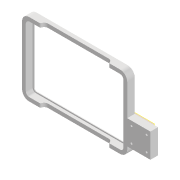
# Autodesk Inventor part: 20_Cube_Insert_Linear_Stage_NEMA11_china_wellplatemount
Saved by Autodesk Inventor 2022 (Build 260153000, 153)
## iProperties
Created: 2022-01-15
Part Number: 20_Cube_Insert_Linear_Stage_NEMA11_china_wellplatemount
Material: Generisch
Document SubType Name: Modeling
Designer: diederichbenedict
Density: 1 g/cm^3
Appearance: Vorgabe
Author: diederichbenedict
Autodesk Inventor part; units mm, degrees
ref_plane "YZ Plane" through (0, 0, 0) normal (1, 0, 0) x (0, 1, 0)
ref_plane "XZ Plane" through (0, 0, 0) normal (0, 1, 0) x (-1, 0, 0)
ref_plane "XY Plane" through (0, 0, 0) normal (0, 0, 1) x (1, 0, 0)
ref_plane "Arbeitsebene1" through (-6.2499, 0, 0) normal (0, 0, 1) x (1, 0, 0)
sketch "Skizze1" plane through (-6.2499, 0, 0) normal (0, 0, 1) x (1, 0, 0)
  line L0 (21.2499, 26.0506) -> (21.2499, 58.2506) projected
  line L1 (21.2499, 58.2506) -> (-8.7501, 58.2506) projected
  line L2 (-8.7501, 58.2506) -> (-8.7501, 26.0506) projected
  line L3 (-8.7501, 26.0506) -> (21.2499, 26.0506) projected
  circle A0 centre (16.2499, 32.1506) radius 1.25 projected
  circle A1 centre (-3.7501, 32.1506) radius 1.25 projected
  circle A2 centre (-3.7501, 52.1506) radius 1.25 projected
  circle A3 centre (16.2499, 52.1506) radius 1.25 projected
  circle A4 centre (13.7499, 38.0506) radius 3.25 projected
  circle A5 centre (13.7499, 46.2506) radius 3.25 projected
  circle A6 centre (-1.2501, 38.0506) radius 3.25 projected
  circle A7 centre (-1.2501, 46.2506) radius 3.25 projected
  line L4 (-67.7501, 103.2266) -> (-67.7501, 101.9266) construction
  line L5 (-18.7501, 103.2266) -> (-67.7501, 103.2266) construction
  arc A8 (-15.2501, 99.7266) -> (-18.7501, 103.2266) centre (-18.7501, 99.7266) ccw construction
  line L6 (-15.2501, 22.1266) -> (-15.2501, 99.7266) construction
  arc A9 (-18.7501, 18.6266) -> (-15.2501, 22.1266) centre (-18.7501, 22.1266) ccw construction
  line L7 (-67.7501, 18.6266) -> (-18.7501, 18.6266) construction
  line L8 (-67.7501, 19.9266) -> (-67.7501, 18.6266) construction
  line L9 (-23.4028, 19.9266) -> (-67.7501, 19.9266) construction
  arc A10 (-23.4028, 19.9266) -> (-21.8472, 20.571) centre (-23.4028, 22.1266) ccw construction
  line L10 (-17.1945, 25.2237) -> (-21.8472, 20.571) construction
  arc A11 (-17.1945, 25.2237) -> (-16.5501, 26.7793) centre (-18.7501, 26.7793) ccw construction
  line L11 (-16.5501, 95.0739) -> (-16.5501, 26.7793) construction
  arc A12 (-16.5501, 95.0739) -> (-17.1945, 96.6296) centre (-18.7501, 95.0739) ccw construction
  line L12 (-21.8472, 101.2823) -> (-17.1945, 96.6296) construction
  arc A13 (-21.8472, 101.2823) -> (-23.4028, 101.9266) centre (-23.4028, 99.7266) ccw construction
  line L13 (-67.7501, 101.9266) -> (-23.4028, 101.9266) construction
  arc A14 (-18.7501, 18.2266) -> (-14.8501, 22.1266) centre (-18.7501, 22.1266) ccw construction
  line L14 (-14.8501, 22.1266) -> (-14.8501, 99.7266) construction
  line L15 (-18.7501, 103.6266) -> (-68.1501, 103.6266) construction
  line L16 (-68.1501, 103.6266) -> (-68.1501, 101.5266) construction
  line L17 (-68.1501, 101.5266) -> (-23.4028, 101.5266) construction
  arc A15 (-22.13, 100.9994) -> (-23.4028, 101.5266) centre (-23.4028, 99.7266) ccw construction
  line L18 (-22.13, 100.9994) -> (-17.4773, 96.3467) construction
  arc A16 (-16.9501, 95.0739) -> (-17.4773, 96.3467) centre (-18.7501, 95.0739) ccw construction
  line L19 (-16.9501, 95.0739) -> (-16.9501, 26.7793) construction
  arc A17 (-17.4773, 25.5065) -> (-16.9501, 26.7793) centre (-18.7501, 26.7793) ccw construction
  line L20 (-17.4773, 25.5065) -> (-22.13, 20.8538) construction
  arc A18 (-23.4028, 20.3266) -> (-22.13, 20.8538) centre (-23.4028, 22.1266) ccw construction
  line L21 (-23.4028, 20.3266) -> (-68.1501, 20.3266) construction
  line L22 (-68.1501, 20.3266) -> (-68.1501, 18.2266) construction
  line L23 (-68.1501, 18.2266) -> (-18.7501, 18.2266) construction
  arc A19 (-18.7501, 18.2266) -> (-14.8501, 22.1266) centre (-18.7501, 22.1266) ccw construction
  line L24 (-14.8501, 22.1266) -> (-14.8501, 99.7266) construction
  arc A20 (-14.8501, 99.7266) -> (-18.7501, 103.6266) centre (-18.7501, 99.7266) ccw construction
  line L25 (-89.5501, 101.9266) -> (-89.5501, 103.2266) construction
  line L26 (-138.8501, 101.9266) -> (-89.5501, 101.9266) construction
  arc A21 (-138.8501, 101.9266) -> (-140.7501, 100.0266) centre (-138.8501, 100.0266) ccw construction
  line L27 (-140.7501, 21.8266) -> (-140.7501, 100.0266) construction
  arc A22 (-140.7501, 21.8266) -> (-138.8501, 19.9266) centre (-138.8501, 21.8266) ccw construction
  line L28 (-89.5501, 19.9266) -> (-138.8501, 19.9266) construction
  line L29 (-89.5501, 18.6266) -> (-89.5501, 19.9266) construction
  line L30 (-138.5501, 18.6266) -> (-89.5501, 18.6266) construction
  arc A23 (-142.0501, 22.1266) -> (-138.5501, 18.6266) centre (-138.5501, 22.1266) ccw construction
  line L31 (-142.0501, 99.7266) -> (-142.0501, 22.1266) construction
  arc A24 (-138.5501, 103.2266) -> (-142.0501, 99.7266) centre (-138.5501, 99.7266) ccw construction
  line L32 (-89.5501, 103.2266) -> (-138.5501, 103.2266) construction
  arc A25 (-138.5501, 103.6266) -> (-142.4501, 99.7266) centre (-138.5501, 99.7266) ccw construction
  line L33 (-142.4501, 99.7266) -> (-142.4501, 22.1266) construction
  arc A26 (-142.4501, 22.1266) -> (-138.5501, 18.2266) centre (-138.5501, 22.1266) ccw construction
  line L34 (-138.5501, 18.2266) -> (-89.1501, 18.2266) construction
  line L35 (-89.1501, 18.2266) -> (-89.1501, 20.3266) construction
  line L36 (-89.1501, 20.3266) -> (-138.8501, 20.3266) construction
  arc A27 (-140.3501, 21.8266) -> (-138.8501, 20.3266) centre (-138.8501, 21.8266) ccw construction
  line L37 (-140.3501, 21.8266) -> (-140.3501, 100.0266) construction
  arc A28 (-138.8501, 101.5266) -> (-140.3501, 100.0266) centre (-138.8501, 100.0266) ccw construction
  line L38 (-138.8501, 101.5266) -> (-89.1501, 101.5266) construction
  line L39 (-89.1501, 101.5266) -> (-89.1501, 103.6266) construction
  line L40 (-89.1501, 103.6266) -> (-138.5501, 103.6266) construction
  line L41 (-68.6501, 104.1266) -> (-18.7501, 104.1266)
  arc A29 (-14.3501, 99.7266) -> (-18.7501, 104.1266) centre (-18.7501, 99.7266) ccw
  line L42 (-14.3501, 99.7266) -> (-14.3501, 22.1266)
  arc A30 (-18.7501, 17.7266) -> (-14.3501, 22.1266) centre (-18.7501, 22.1266) ccw
  line L43 (-18.7501, 17.7266) -> (-68.6501, 17.7266)
  line L44 (-68.6501, 17.7266) -> (-68.6501, 20.8266)
  line L45 (-68.6501, 20.8266) -> (-23.4028, 20.8266)
  arc A31 (-23.4028, 20.8266) -> (-22.4836, 21.2074) centre (-23.4028, 22.1266) ccw
  line L46 (-22.4836, 21.2074) -> (-17.8309, 25.8601)
  arc A32 (-17.8309, 25.8601) -> (-17.4501, 26.7793) centre (-18.7501, 26.7793) ccw
  line L47 (-17.4501, 26.7793) -> (-17.4501, 95.0739)
  arc A33 (-17.4501, 95.0739) -> (-17.8309, 95.9932) centre (-18.7501, 95.0739) ccw
  line L48 (-17.8309, 95.9932) -> (-22.4836, 100.6459)
  arc A34 (-22.4836, 100.6459) -> (-23.4028, 101.0266) centre (-23.4028, 99.7266) ccw
  line L49 (-23.4028, 101.0266) -> (-68.6501, 101.0266)
  line L50 (-68.6501, 101.0266) -> (-68.6501, 104.1266)
  arc A35 (-138.5501, 104.1266) -> (-142.9501, 99.7266) centre (-138.5501, 99.7266) ccw
  line L51 (-142.9501, 99.7266) -> (-142.9501, 22.1266)
  arc A36 (-142.9501, 22.1266) -> (-138.5501, 17.7266) centre (-138.5501, 22.1266) ccw
  line L52 (-138.5501, 17.7266) -> (-88.6501, 17.7266)
  line L53 (-88.6501, 17.7266) -> (-88.6501, 20.8266)
  line L54 (-88.6501, 20.8266) -> (-138.8501, 20.8266)
  arc A37 (-139.8501, 21.8266) -> (-138.8501, 20.8266) centre (-138.8501, 21.8266) ccw
  line L55 (-139.8501, 21.8266) -> (-139.8501, 100.0266)
  arc A38 (-138.8501, 101.0266) -> (-139.8501, 100.0266) centre (-138.8501, 100.0266) ccw
  line L56 (-138.8501, 101.0266) -> (-88.6501, 101.0266)
  line L57 (-88.6501, 101.0266) -> (-88.6501, 104.1266)
  line L58 (-88.6501, 104.1266) -> (-138.5501, 104.1266)
  line L59 (-68.6501, 104.1266) -> (-88.6501, 104.1266)
  line L60 (-88.6501, 17.7266) -> (-68.6501, 17.7266)
  line L61 (-94.9, 12.7266) -> (-138.5501, 12.7266)
  arc A39 (-147.9501, 22.1266) -> (-138.5501, 12.7266) centre (-138.5501, 22.1266) ccw
  line L62 (-147.9501, 22.1266) -> (-147.9501, 99.7266)
  arc A40 (-138.5501, 109.1266) -> (-147.9501, 99.7266) centre (-138.5501, 99.7266) ccw
  line L63 (-138.5501, 109.1266) -> (-94.9, 109.1266)
  line L64 (-74.9, 12.7266) -> (-18.7501, 12.7266)
  arc A41 (-18.7501, 12.7266) -> (-9.3501, 22.1266) centre (-18.7501, 22.1266) ccw
  line L65 (-9.3501, 22.1266) -> (-9.3501, 99.7266)
  arc A42 (-9.3501, 99.7266) -> (-18.7501, 109.1266) centre (-18.7501, 99.7266) ccw
  line L66 (-18.7501, 109.1266) -> (-74.9, 109.1266)
  line L67 (-94.9, 12.7266) -> (-74.9, 12.7266)
  line L68 (-74.9, 109.1266) -> (-94.9, 109.1266)
  line L69 (-8.7501, 58.2506) -> (-9.3501, 58.2506)
  line L70 (-8.7501, 26.0506) -> (-9.3501, 26.0506)
  point P0 (6.2499, 0)
  point P1 (-12.4751, 58.2506)
  point P2 (-12.4751, 26.0506)
  point P3 (-12.4751, 26.0506)
  dimension "d0" = 0
  dimension "d1" = 0
  dimension "d2" = 0.5
  dimension "d3" = 0.5
  dimension "d4" = 5
  dimension "d5" = 5
  constraints: 96 end point, 48 point on circle, 24 centre point, 2 point on line, 1 parallel, 1 perpendicular, 60 other
  measures "d0" distance between parallel lines of L40 L15
  measures "d1" distance between parallel lines of L24 L14
  measures "d2" distance between parallel lines of L15 L41
  measures "d3" distance between parallel lines of L40 L58
  measures "d4" distance between parallel lines of L52 L61
  measures "d5" distance between parallel lines of L43 L64
extrude "Extrusion1" add sketch "Skizze1" along normal blind 10 contours L3 L2 L1 L0 | L70 L65 L69 L2 | L65 A41 L64 L67 L61 A39 L62 A40 L63 L68 L66 A42 | A4 | A5 | A6 | A7
sketch "Skizze3" plane through (-6.2499, 0, 0) normal (0, 0, -1) x (-1, 0, 0)
  line L0 (9.3501, 26.0506) -> (-21.2499, 26.0506) projected
  line L1 (9.3501, 22.1266) -> (9.3501, 26.0506) projected
  arc A0 (9.3501, 22.1266) -> (18.7501, 12.7266) centre (18.7501, 22.1266) ccw projected
  line L2 (138.5501, 12.7266) -> (18.7501, 12.7266) projected
  arc A1 (138.5501, 12.7266) -> (147.9501, 22.1266) centre (138.5501, 22.1266) ccw projected
  line L3 (147.9501, 99.7266) -> (147.9501, 22.1266) projected
  arc A2 (147.9501, 99.7266) -> (138.5501, 109.1266) centre (138.5501, 99.7266) ccw projected
  line L4 (18.7501, 109.1266) -> (138.5501, 109.1266) projected
  arc A3 (18.7501, 109.1266) -> (9.3501, 99.7266) centre (18.7501, 99.7266) ccw projected
  line L5 (9.3501, 58.2506) -> (9.3501, 99.7266) projected
  line L6 (-21.2499, 58.2506) -> (9.3501, 58.2506) projected
  line L7 (-21.2499, 26.0506) -> (-21.2499, 58.2506) projected
  circle A4 centre (-16.2499, 32.1506) radius 1.25 projected
  circle A5 centre (3.7501, 32.1506) radius 1.25 projected
  circle A6 centre (3.7501, 52.1506) radius 1.25 projected
  circle A7 centre (-16.2499, 52.1506) radius 1.25 projected
  line L8 (18.7501, 17.7266) -> (138.5501, 17.7266) projected
  arc A8 (14.3501, 22.1266) -> (18.7501, 17.7266) centre (18.7501, 22.1266) ccw projected
  line L9 (14.3501, 99.7266) -> (14.3501, 22.1266) projected
  arc A9 (18.7501, 104.1266) -> (14.3501, 99.7266) centre (18.7501, 99.7266) ccw projected
  line L10 (138.5501, 104.1266) -> (18.7501, 104.1266) projected
  arc A10 (142.9501, 99.7266) -> (138.5501, 104.1266) centre (138.5501, 99.7266) ccw projected
  line L11 (142.9501, 22.1266) -> (142.9501, 99.7266) projected
  arc A11 (138.5501, 17.7266) -> (142.9501, 22.1266) centre (138.5501, 22.1266) ccw projected
  arc A12 (141.4501, 99.7266) -> (138.5501, 102.6266) centre (138.5501, 99.7266) ccw
  line L12 (138.5501, 102.6266) -> (18.7501, 102.6266)
  arc A13 (18.7501, 102.6266) -> (15.8501, 99.7266) centre (18.7501, 99.7266) ccw
  line L13 (15.8501, 99.7266) -> (15.8501, 22.1266)
  arc A14 (15.8501, 22.1266) -> (18.7501, 19.2266) centre (18.7501, 22.1266) ccw
  line L14 (18.7501, 19.2266) -> (138.5501, 19.2266)
  arc A15 (138.5501, 19.2266) -> (141.4501, 22.1266) centre (138.5501, 22.1266) ccw
  line L15 (141.4501, 22.1266) -> (141.4501, 99.7266)
  point P0 (-6.2499, 0)
  dimension "d11" = 1.5
  constraints: 8 end point, 8 point on circle, 4 centre point, 7 other
  measures "d11" distance between parallel lines of L11 L15
extrude "Extrusion3" add sketch "Skizze3" against normal blind 1 contours A8 L9 A9 L10 A10 L11 A11 L8
sketch "Skizze4" plane through (-144.8, 12.7266, 0) normal (0, -1, 0) x (1, 0, 0)
  line L0 (0, 10) -> (119.8, 10) projected
  line L1 (19.9, 10) -> (99.9, 10) construction
  line L2 (0, 10) -> (119.8, 10) projected
  line L3 (19.9, 7.5) -> (99.9, 7.5)
  line L4 (99.9, 12.5) -> (19.9, 12.5)
  arc A0 (19.9, 12.5) -> (19.9, 7.5) centre (19.9, 10) ccw
  arc A1 (99.9, 7.5) -> (99.9, 12.5) centre (99.9, 10) ccw
  point P0 (144.8, 0)
  point P1 (59.9, 10)
  point P2 (102.4, 10)
  point P3 (17.4, 10)
  dimension "d14" = 40
  dimension "d18" = 5
  constraints: 8 end point, 4 point on circle, 4 tangent, 2 centre point, 2 midpoint, 1 parallel, 1 point on line
  measures "d14" distance of point (59.9, 10) L1.end
  measures "d18" distance between parallel lines of L3 L4
extrude "Extrusion4" cut sketch "Skizze4" against normal through all contours L0 A1 L3 A0
fillet "Rundung1" radius 2 4 edges at (-127.4, 15.2266, 10) (-127.4, 106.6266, 10) (-42.4, 106.6266, 10) (-42.4, 15.2266, 10)
